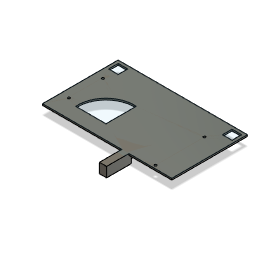
Hopper Rest (Autodesk Fusion 360 design; units mm, degrees)
Autodesk Fusion 360 part; units mm, degrees
sketch "Sketch1" plane through (0, 111.6779, 0) normal (0, 1, 0) x (-1, 0, 0)
  arc A0 (21.4161, -39.9724) -> (59.9595, -1.429) centre (19.9851, 0.002) ccw
  line L0 (21.4161, -39.9724) -> (21.4161, -1.429)
  line L1 (21.4161, -1.429) -> (59.9595, -1.429)
  arc A1 (16.4161, -44.8563) -> (64.8434, 3.571) centre (19.9851, 0.002) ccw
  line L2 (64.8434, 3.571) -> (16.4161, 3.571)
  line L3 (16.4161, 3.571) -> (16.4161, -44.8563)
  line L4 (-32.85, 23.15) -> (-32.85, -19.15)
  line L5 (-32.85, -19.15) -> (-32.85, -36.15)
  line L6 (-32.85, -19.15) -> (-32.85, 25.85)
  line L7 (-32.85, -36.15) -> (-44.5067, -36.15)
  line L8 (-44.5067, -36.15) -> (-44.5067, 33.5264)
  line L9 (-44.5067, 33.5264) -> (-32.85, 33.5264)
  line L10 (-32.85, 33.5264) -> (-32.85, -36.15)
  dimension "d193" = 17
  dimension "d194" = 45
  constraint coincident L4.end L5.start
  constraint parallel L4 L5
  constraint parallel L4 L6
  constraint horizontal L7
  constraint vertical L8
  constraint horizontal L9
  constraint vertical L10
  measures "d193" distance of L4.end L5.end
  measures "d194" distance of L4.end L6.end
extrude "Extrude1" add sketch "Sketch1" along normal blind 9.1 contours L4 L5 L6 L7 L8 L9 L10
sketch "Sketch2" plane through (0, 111.6779, 0) normal (0, -1, 0) x (1, 0, 0)
  line L0 (44.5067, 33.5264) -> (32.85, 33.5264)
  line L1 (32.85, 33.5264) -> (32.85, -36.15)
  line L2 (32.85, -36.15) -> (44.5067, -36.15)
  line L3 (44.5067, -36.15) -> (44.5067, 33.5264)
  line L4 (32.85, 33.5264) -> (44.5067, 33.5264)
  line L5 (44.5067, 33.5264) -> (44.5067, 23.2787)
  line L6 (44.5067, 23.2787) -> (32.85, 23.2787)
  line L7 (32.85, 23.2787) -> (32.85, 33.5264)
  line L8 (44.5067, -36.15) -> (32.85, -36.15)
  line L9 (32.85, -36.15) -> (32.85, -19.2266)
  line L10 (32.85, -19.2266) -> (44.5067, -19.2266)
  line L11 (44.5067, -19.2266) -> (44.5067, -36.15)
  constraint horizontal L4
  constraint vertical L5
  constraint horizontal L6
  constraint vertical L7
  constraint coincident L3 L5.end
  constraint coincident L0.end L1.start
  constraint horizontal L8
  constraint vertical L9
  constraint horizontal L10
  constraint vertical L11
  constraint coincident L1 L9.end
  constraint coincident L2.end L3.start
extrude "Extrude2" add sketch "Sketch2" along normal blind 7 contours L0 L1 L3 L4 L5 L6 L7 | L1 L2 L3 L8 L9 L10 L11
sketch "Sketch3" plane through (0, 120.7779, 0) normal (0, 1, 0) x (-1, 0, 0)
  line L0 (-32.85, 33.5264) -> (-44.5067, 33.5264)
  line L1 (-44.5067, 33.5264) -> (-44.5067, -36.15)
  line L2 (-44.5067, -36.15) -> (-32.85, -36.15)
  line L3 (-32.85, -36.15) -> (-32.85, 33.5264)
  line L4 (16.4161, 3.571) -> (16.4161, -44.8563)
  arc A0 (16.4161, -44.8563) -> (64.8434, 3.571) centre (19.9851, 0.002) ccw
  line L5 (64.8434, 3.571) -> (16.4161, 3.571)
  line L6 (16.4161, 3.571) -> (64.8434, 3.571) construction
  line L7 (16.4161, 3.571) -> (16.4161, -44.8563) construction
  line L8 (16.4161, 3.571) -> (16.4161, -44.8563) construction
  line L9 (75.6661, -90.679) -> (90.9161, -90.679) construction
  line L10 (90.9161, -90.679) -> (90.9161, -75.429) construction
  line L11 (64.8434, 3.571) -> (16.4161, 3.571) construction
  line L12 (90.9161, -90.679) -> (90.9161, -75.429) construction
  line L13 (-109.3339, -75.429) -> (-109.3339, -90.679) construction
  line L14 (16.0661, 3.921) -> (16.0661, -45.1784)
  arc A1 (16.0661, -45.1784) -> (65.1655, 3.921) centre (19.9851, 0.002) ccw
  line L15 (16.0661, 3.921) -> (65.1655, 3.921)
  line L16 (-109.3339, -90.679) -> (-109.3339, -75.429)
  line L17 (90.9161, 22.2835) -> (90.9161, -90.679)
  line L18 (-114.3339, -95.679) -> (-114.3339, 27.2835)
  line L19 (-114.3339, 27.2835) -> (95.9161, 27.2835)
  line L20 (95.9161, 27.2835) -> (95.9161, -95.679)
  line L21 (95.9161, -95.679) -> (-114.3339, -95.679)
  line L22 (90.9161, -90.679) -> (75.9161, -90.679)
  line L23 (75.9161, -90.679) -> (75.9161, -75.679)
  line L24 (75.9161, -75.679) -> (90.9161, -75.679)
  line L25 (90.9161, -75.679) -> (90.9161, -90.679)
  line L26 (-109.3339, -90.679) -> (-94.3339, -90.679)
  line L27 (-94.3339, -90.679) -> (-94.3339, -75.679)
  line L28 (-94.3339, -75.679) -> (-109.3339, -75.679)
  line L29 (-109.3339, -75.679) -> (-109.3339, -90.679)
  line L30 (-109.5839, -90.929) -> (-94.0839, -90.929)
  line L31 (-94.0839, -90.929) -> (-94.0839, -75.429)
  line L32 (-94.0839, -75.429) -> (-109.5839, -75.429)
  line L33 (-109.5839, -75.429) -> (-109.5839, -90.929)
  line L34 (91.1661, -90.929) -> (75.6661, -90.929)
  line L35 (75.6661, -90.929) -> (75.6661, -75.429)
  line L36 (75.6661, -75.429) -> (91.1661, -75.429)
  line L37 (91.1661, -75.429) -> (91.1661, -90.929)
  line L38 (90.9161, -90.679) -> (75.6661, -90.679) construction
  line L39 (-94.0839, -90.679) -> (-109.3339, -90.679) construction
  line L40 (-109.3339, -90.679) -> (-94.0839, -90.679) construction
  line L41 (75.6661, -90.679) -> (90.9161, -90.679) construction
  line L42 (90.9161, -90.679) -> (75.6661, -90.679)
  line L43 (-94.0839, -90.679) -> (-109.3339, -90.679)
  dimension "d201" = 200.25
  dimension "d202" = 0.35
  dimension "d204" = 15
  dimension "d205" = 15
  dimension "d206" = 15
  dimension "d207" = 15
  dimension "d208" = 0.25
  dimension "d209" = -0.25
  constraint coincident L4.start L5.end
  constraint perpendicular L4 L6
  constraint perpendicular L5 L7
  constraint perpendicular L8 L9
  constraint parallel L8 L10
  constraint parallel L9 L11
  constraint perpendicular L10 L38
  constraint perpendicular L12 L40
  constraint parallel L12 L13
  constraint horizontal L42
  constraint vertical L16
  constraint vertical L17
  constraint horizontal L22
  constraint vertical L23
  constraint horizontal L24
  constraint vertical L25
  constraint horizontal L26
  constraint vertical L27
  constraint horizontal L28
  constraint vertical L29
  constraint coincident L32 L13.start
  constraint parallel L16 L18
  constraint parallel L17 L20
  constraint parallel L21 L42
  constraint coincident L35 L9.start
  constraint coincident L31 L39.start
  constraint collinear L38 L39
  constraint collinear L40 L41
  constraint collinear L42 L43
  constraint coincident L36 L10.end
  measures "d201" distance of L9.end L13.end
  measures "d204" distance of L9.end L22.end
  measures "d205" distance of L9.end L24.end
  measures "d206" distance of L13.end L26.end
  measures "d207" distance of L13.end L28.end
extrude "Extrude3" add sketch "Sketch3" against normal blind 2.5 contours L1 L2 L3 L18 L19 L20 L21
sketch "Sketch4" plane through (0, 120.7779, 0) normal (0, 1, 0) x (-1, 0, 0)
  line L0 (-109.5839, -90.929) -> (-109.5839, -75.429)
  line L1 (-109.5839, -75.429) -> (-94.0839, -75.429)
  line L2 (-94.0839, -75.429) -> (-94.0839, -90.929)
  line L3 (-94.0839, -90.929) -> (-109.5839, -90.929)
  arc A0 (16.0661, -45.1784) -> (65.1655, 3.921) centre (19.9851, 0.002) ccw
  line L4 (16.0661, -45.1784) -> (16.0661, 3.921)
  line L5 (16.0661, 3.921) -> (65.1655, 3.921)
  line L6 (75.6661, -75.429) -> (91.1661, -75.429)
  line L7 (91.1661, -75.429) -> (91.1661, -90.929)
  line L8 (91.1661, -90.929) -> (75.6661, -90.929)
  line L9 (75.6661, -90.929) -> (75.6661, -75.429)
  line L10 (-32.85, 33.5264) -> (-44.5067, 33.5264)
  line L11 (-44.5067, 33.5264) -> (-44.5067, 27.2835)
  line L12 (-44.5067, 27.2835) -> (-114.3339, 27.2835)
  line L13 (-114.3339, 27.2835) -> (-114.3339, -95.679)
  line L14 (-114.3339, -95.679) -> (95.9161, -95.679)
  line L15 (95.9161, -95.679) -> (95.9161, 27.2835)
  line L16 (95.9161, 27.2835) -> (-32.85, 27.2835)
  line L17 (-32.85, 27.2835) -> (-32.85, 33.5264)
sketch "Sketch5" plane through (0, 118.2779, 0) normal (0, -1, 0) x (1, 0, 0)
  line L0 (-91.1661, -75.429) -> (-75.6661, -75.429)
  line L1 (-75.6661, -75.429) -> (-75.6661, -90.929)
  line L2 (-75.6661, -90.929) -> (-91.1661, -90.929)
  line L3 (-91.1661, -90.929) -> (-91.1661, -75.429)
  arc A0 (-65.1655, 3.921) -> (-16.0661, -45.1784) centre (-19.9851, 0.002) ccw
  line L4 (-65.1655, 3.921) -> (-16.0661, 3.921)
  line L5 (-16.0661, 3.921) -> (-16.0661, -45.1784)
  line L6 (109.5839, -75.429) -> (109.5839, -90.929)
  line L7 (109.5839, -90.929) -> (94.0839, -90.929)
  line L8 (94.0839, -90.929) -> (94.0839, -75.429)
  line L9 (94.0839, -75.429) -> (109.5839, -75.429)
  line L10 (-95.9161, 27.2835) -> (-95.9161, -95.679)
  line L11 (-95.9161, -95.679) -> (114.3339, -95.679)
  line L12 (114.3339, -95.679) -> (114.3339, 27.2835)
  line L13 (114.3339, 27.2835) -> (44.5067, 27.2835)
  line L14 (44.5067, 27.2835) -> (44.5067, -36.15)
  line L15 (44.5067, -36.15) -> (32.85, -36.15)
  line L16 (32.85, -36.15) -> (32.85, 27.2835)
  line L17 (32.85, 27.2835) -> (-95.9161, 27.2835)
  circle A1 centre (-82.5, -2.5) radius 1.5
  circle A2 centre (-82.5, -57.5) radius 1.5
  circle A3 centre (82.6, -57.5) radius 1.5
  circle A4 centre (82.625, 22.0438) radius 1.5
  circle A5 centre (-82.5, -2.5) radius 1.85
  circle A6 centre (-82.5, -57.5) radius 1.85
  circle A7 centre (82.6, -57.5) radius 1.85
  circle A8 centre (82.625, 22.0438) radius 1.85
  dimension "d221" = 0.35
  dimension "d222" = 0.35
  dimension "d223" = 0.35
  dimension "d224" = 0.35
extrude "Extrude4" cut sketch "Sketch5" against normal blind 3 contours A1 | A2 | A3 | A4 | A5 | A6 | A7 | A8
extrude "Extrude5" add 1 faces at (40.6211, 110.0446, 33.5264) along direction (0, 0, 1) blind 30
